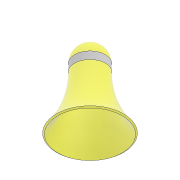
# Autodesk Inventor part: cock
Saved by Autodesk Inventor 2021 (Build 250183000, 183)
## iProperties
Created: 2021-07-23
Part Number: cock
Material: Generic
Document SubType Name: Modeling
Designer: user
Density: 1 g/cm^3
Appearance: White
Author: user
Autodesk Inventor part; units mm, degrees
ref_plane "YZ Plane" through (0, 0, 0) normal (1, 0, 0) x (0, 1, 0)
ref_plane "XZ Plane" through (0, 0, 0) normal (0, 1, 0) x (-1, 0, 0)
ref_plane "XY Plane" through (0, 0, 0) normal (0, 0, 1) x (1, 0, 0)
sketch "Sketch1" plane through (0, 0, 0) normal (0, 1, 0) x (-1, 0, 0)
  arc A0 (31.75, 0) -> (-31.75, 0) centre (0, 0) ccw
  line L0 (31.75, 0) -> (-31.75, 0)
  line L1 (44.45, 0) -> (-44.45, 0) projected
  dimension "d0" = 31.75
  constraints: 2 end point, 2 point on circle, 1 centre point, 1 coincident, 1 horizontal
  measures "d0" radius of A0
revolve "Revolution1" add sketch "Sketch1" angle 180 about axis through (-10, 0, 0) along (-1, 0, 0)
sketch "Sketch2" plane through (0, 0, 0) normal (0, -1, 0) x (1, 0, 0)
  circle A0 centre (0, 0) radius 31.75
  constraints: 1 centre point, 1 coincident
extrude "Extrusion1" add sketch "Sketch2" along normal blind 15.24
sketch "Sketch3" plane through (0, 0, 0) normal (1, 0, 0) x (0, 1, 0)
  line L0 (-15.24, 31.75) -> (-15.24, -31.75) projected
  line L1 (-15.24, -31.75) -> (-15.24, 0)
  line L2 (-15.24, -31.75) -> (0, -31.75)
  line L3 (0, -31.75) -> (-15.24, -31.75) projected
  arc A0 (-15.24, -31.75) -> (-124.216, -69.0613) centre (-15.24, -209.55) ccw
  arc A1 (-15.24, -28.3717) -> (-126.2866, -66.392) centre (-15.24, -209.55) ccw
  line L4 (-124.216, -69.0613) -> (-126.2866, -66.392)
  line L5 (-15.24, -28.3717) -> (-15.24, -31.75)
  line L6 (0, 31.75) -> (0, -31.75) projected
  line L7 (-161.6909, 0) -> (63.9902, 0) projected
  point P0 (0, 0)
  point P1 (-116.84, 0)
  point P2 (-15.24, -28.3717)
  dimension "d4" = 101.6
  dimension "d5" = 177.8
  constraints: 8 end point, 4 point on circle, 2 centre point, 1 collinear, 1 midpoint, 1 parallel, 1 point on line, 1 tangent
  measures "d4" distance of point (-116.84, 0) L1.end
  measures "d5" radius of A0
sketch "Sketch4" plane through (0, 0, 0) normal (1, 0, 0) x (0, 1, 0)
  point P0 (0, 0)
revolve "Revolution2" add sketch "Sketch3" angle 360 about axis through (0, -10, 0) along (0, 1, 0) contours L0 A0 L4 A1
sketch "Sketch5" plane through (0, -15.24, 0) normal (0, -1, 0) x (1, 0, 0)
  circle A0 centre (0, 0) radius 28.3717
  constraints: 1 centre point, 1 coincident
sketch "Sketch8" plane through (0, 0, 0) normal (1, 0, 0) x (0, 1, 0)
  point P0 (0, 0)
sketch "Sketch9" plane through (0, 0, 0) normal (0, 1, 0) x (-1, 0, 0)
  circle A0 centre (0, 0) radius 28.5845
  circle A1 centre (0, 0) radius 28.5845
  circle A2 centre (0, 0) radius 28.5845
  constraints: 3 centre point, 3 coincident
body "Solid1"
